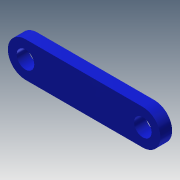
# Autodesk Inventor part: tahlo5
Saved by Autodesk Inventor 2013 (Build 170138000, 138)
## iProperties
Created: 2013-02-02
Part Number: tahlo5
Material: Generic
Document SubType Name: Modeling
Designer: idle-rug
Density: 1 g/cm^3
Author: idle-rug
Autodesk Inventor part; units mm, degrees
ref_plane "YZ Plane" through (0, 0, 0) normal (1, 0, 0) x (0, 1, 0)
ref_plane "XZ Plane" through (0, 0, 0) normal (0, 1, 0) x (-1, 0, 0)
ref_plane "XY Plane" through (0, 0, 0) normal (0, 0, 1) x (1, 0, 0)
sketch "Sketch1" plane through (0, 0, 0) normal (0, 1, 0) x (-1, 0, 0)
  line L0 (-10, -3) -> (10, -3)
  line L1 (10, -3) -> (10, 3)
  line L2 (10, 3) -> (-10, 3)
  line L3 (-10, 3) -> (-10, -3)
  line L4 (-10, -3) -> (10, 3) construction
  line L5 (10, -3) -> (-10, 3) construction
  circle A0 centre (10, 0) radius 3
  circle A1 centre (-10, 0) radius 3
  point P0 (0, 0)
  dimension "d0" = 20
  dimension "d1" = 6
  dimension "d2" = 6
  dimension "d3" = 6
  constraints: 12 end point, 4 midpoint, 2 centre point, 2 parallel, 1 horizontal, 1 perpendicular
  measures "d0" distance of L2.end L1.end
  measures "d1" distance of L1.end L0.end
  measures "d2" diameter of A0
  measures "d3" diameter of A1
extrude "Extrusion1" add sketch "Sketch1" along normal blind 2
sketch "Sketch2" plane through (0, 2, 0) normal (0, 1, 0) x (1, 0, 0)
  arc A0 (10, -3) -> (10, 3) centre (10, 0) ccw projected
  arc A1 (-10, 3) -> (-10, -3) centre (-10, 0) ccw projected
  circle A2 centre (-10, 0) radius 1
  circle A3 centre (10, 0) radius 1.5
  circle A4 centre (-10, 0) radius 1.5
  point P0 (0, 0)
  dimension "d6" = 2
  dimension "d7" = 3
  dimension "d8" = 3
  constraints: 3 centre point, 3 coincident
  measures "d6" diameter of A2
  measures "d7" diameter of A3
  measures "d8" diameter of A4
extrude "Extrusion2" cut sketch "Sketch2" against normal blind 2 contours A2 | A3 | A4
body "Solid1"
